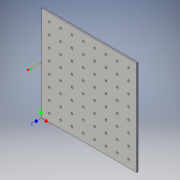
# Autodesk Inventor part: Soldering-guide
Saved by Autodesk Inventor 2016 (Build 200138000, 138)
## iProperties
Created: 2018-02-05
Part Number: Soldering-guide
Material: Generic
Document SubType Name: Modeling
Designer: Nuwan
Density: 1 g/cm^3
Appearance: Default
Author: Nuwan
Autodesk Inventor part; units mm, degrees
ref_plane "YZ Plane" through (0, 0, 0) normal (1, 0, 0) x (0, 1, 0)
ref_plane "XZ Plane" through (0, 0, 0) normal (0, 1, 0) x (-1, 0, 0)
ref_plane "XY Plane" through (0, 0, 0) normal (0, 0, 1) x (1, 0, 0)
sketch "Sketch3" plane through (0, 0, 0) normal (0, 0, 1) x (1, 0, 0)
  line L0 (0, 0) -> (150, 0)
  line L1 (150, 0) -> (150, 150)
  line L2 (150, 150) -> (0, 150)
  line L3 (0, 150) -> (0, 0)
  dimension "d0" = 150
  dimension "d1" = 150
  constraints: 8 end point, 2 parallel, 1 horizontal, 1 perpendicular
  measures "d0" distance of L0.start L0.end
  measures "d1" distance of L2.end L0.start
extrude "Extrusion1" add sketch "Sketch3" along normal blind 3
sketch "Sketch5" plane through (0, 0, 3) normal (0, 0, 1) x (1, 0, 0)
  line L0 (0, 0) -> (150, 0) projected
  line L1 (150, 0) -> (150, 150) projected
  line L2 (150, 150) -> (0, 150) projected
  line L3 (0, 150) -> (0, 0) projected
  line L4 (12, 150) -> (12, 0) construction
  line L5 (0, 138) -> (150, 138) construction
  circle A0 centre (12, 138) radius 1.5
  dimension "d15" = 12
  dimension "d16" = 12
  dimension "d17" = 3
  constraints: 6 point on line, 4 end point, 2 perpendicular, 1 centre point
  measures "d15" distance between parallel lines of L2 L5
  measures "d16" distance between parallel lines of L3 L4
  measures "d17" diameter of A0
extrude "Extrusion2" cut sketch "Sketch5" against normal blind 3 contours A0
pattern_linear "Rectangular Pattern1" count 8 spacing 18 along (1, 0, 0) count 8 spacing 18 along (0, -1, 0) of "Extrusion2"
body "Solid1"
